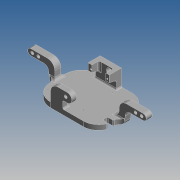
# Autodesk Inventor part: I006
Saved by Autodesk Inventor 2017 (Build 210142000, 142)
## iProperties
Created: 2018-10-19
Part Number: I006
Material: ABS
Document SubType Name: Modeling
Designer: Gilles Mottiez
Density: 1.06 g/cm^3
Appearance: Par défaut
Description: Plateforme mobile
Mass: 94.2161 g
Surface Area: 294.78 cm^2
Volume: 88.8831 cm^3
Author: Gilles Mottiez
Autodesk Inventor part; units mm, degrees
ref_plane "YZ Plane" through (0, 0, 0) normal (1, 0, 0) x (0, 1, 0)
ref_plane "XZ Plane" through (0, 0, 0) normal (0, 1, 0) x (-1, 0, 0)
ref_plane "XY Plane" through (0, 0, 0) normal (0, 0, 1) x (1, 0, 0)
sketch "Sketch1" plane through (0, 0, 0) normal (0, 0, 1) x (1, 0, 0)
  line L0 (0, 0) -> (106, 0)
  line L1 (106, 0) -> (106, -80)
  line L2 (106, -80) -> (0, -80)
  line L3 (0, -80) -> (0, 0)
  dimension "d0" = 106
  dimension "d1" = 80
  constraints: 8 end point, 2 parallel, 1 horizontal, 1 perpendicular
  measures "d0" distance of L0.start L0.end
  measures "d1" distance of L2.end L0.start
extrude "Extrusion1" add sketch "Sketch1" along normal blind 8
sketch "Esquisse2" plane through (0, 0, 8) normal (0, 0, 1) x (1, 0, 0)
  line L0 (106, 0) -> (0, 0) construction
  line L1 (0, 0) -> (0, -80) construction
  line L2 (0, -80) -> (106, -80) construction
  line L3 (106, -80) -> (106, 0) construction
  line L4 (8, -15.5) -> (66, -15.5) construction
  line L5 (66, -15.5) -> (66, -64.5) construction
  line L6 (66, -64.5) -> (8, -64.5) construction
  line L7 (8, -64.5) -> (8, -15.5) construction
  line L8 (0, -40) -> (106, -40) construction
  dimension "d4" = 58
  dimension "d5" = 49
  dimension "d6" = 8
  constraints: 10 end point, 4 coincident, 2 midpoint, 2 parallel, 1 horizontal, 1 perpendicular, 1 other
  measures "d4" distance of L4.start L4.end
  measures "d5" distance of L4.end L5.end
  measures "d6" distance between parallel lines of L1 L7
hole "Perçage1" at (8, -15.5, 8) at (8, -64.5, 8) at (66, -64.5, 8) at (66, -15.5, 8) direction (0, 0, -1) diameter 2 end through all
sketch "Esquisse3" plane through (106, -80, 0) normal (1, 0, 0) x (0, 0, -1)
  line L0 (0, 80) -> (0, 0) construction
  line L1 (0, 80) -> (-8, 80) construction
  line L2 (-8, 0) -> (-8, 80) construction
  line L3 (0, 0) -> (-8, 0) construction
  line L4 (-8, 40) -> (0, 40) construction
  line L5 (0, 45) -> (-33, 45)
  line L6 (-33, 45) -> (-33, 35)
  line L7 (-33, 35) -> (0, 35)
  line L8 (0, 35) -> (0, 45)
  dimension "d14" = 33
  dimension "d15" = 10
  constraints: 10 end point, 2 midpoint, 2 parallel, 1 horizontal, 1 perpendicular, 1 point on line, 1 other
  measures "d14" distance of L7.end L6.end
  measures "d15" distance of L5.end L6.end
extrude "Extrusion2" add sketch "Esquisse3" along normal blind 10
sketch "Esquisse4" plane through (0, -80, 0) normal (-1, 0, 0) x (0, 0, 1)
  line L0 (0, 0) -> (0, 80) construction
  line L1 (0, 0) -> (8, 0) construction
  line L2 (8, 80) -> (8, 0) construction
  line L3 (0, 80) -> (8, 80) construction
  line L4 (8, 40) -> (0, 40) construction
  line L5 (0, 45) -> (33, 45)
  line L6 (33, 45) -> (33, 35)
  line L7 (33, 35) -> (0, 35)
  line L8 (0, 35) -> (0, 45)
  dimension "d18" = 33
  dimension "d19" = 10
  constraints: 10 end point, 2 midpoint, 2 parallel, 1 horizontal, 1 perpendicular, 1 point on line, 1 other
  measures "d18" distance of L6.end L7.end
  measures "d19" distance of L5.end L6.end
extrude "Extrusion3" add sketch "Esquisse4" along normal blind 10
sketch "Esquisse5" plane through (-10, -80, 0) normal (-1, 0, 0) x (0, 0, 1)
  line L0 (33, 45) -> (0, 45) construction
  line L1 (0, 45) -> (0, 35) construction
  line L2 (0, 35) -> (33, 35) construction
  line L3 (33, 35) -> (33, 45) construction
  line L4 (33, 45) -> (23, 45)
  line L5 (23, 45) -> (23, 35)
  line L6 (23, 35) -> (33, 35)
  line L7 (33, 35) -> (33, 45)
  point P0 (0, 80)
  dimension "d22" = 10
  constraints: 8 end point, 2 parallel, 1 horizontal, 1 perpendicular, 1 point on line
  measures "d22" distance of L6.end L5.end
extrude "Extrusion4" add sketch "Esquisse5" along normal blind 34.5
sketch "Esquisse6" plane through (116, -80, 0) normal (1, 0, 0) x (0, 0, -1)
  line L0 (0, 45) -> (-33, 45) construction
  line L1 (-33, 45) -> (-33, 35) construction
  line L2 (-33, 35) -> (0, 35) construction
  line L3 (0, 35) -> (0, 45) construction
  line L4 (-33, 35) -> (-23, 35)
  line L5 (-23, 35) -> (-23, 45)
  line L6 (-23, 45) -> (-33, 45)
  line L7 (-33, 45) -> (-33, 35)
  point P0 (0, 80)
  dimension "d25" = 10
  constraints: 8 end point, 2 parallel, 1 horizontal, 1 perpendicular, 1 point on line
  measures "d25" distance of L6.end L5.end
extrude "Extrusion5" add sketch "Esquisse6" along normal blind 34.5
sketch "Esquisse7" plane through (0, -80, 0) normal (0, -1, 0) x (1, 0, 0)
  line L0 (106, 0) -> (0, 0) construction
  line L1 (106, 0) -> (106, 8) construction
  line L2 (0, 8) -> (106, 8) construction
  line L3 (0, 0) -> (0, 8) construction
  line L4 (53, 8) -> (53, 0) construction
  line L5 (28, 8) -> (63, 8) construction
  line L6 (63, 8) -> (63, 28) construction
  line L7 (63, 28) -> (28, 28) construction
  line L8 (28, 28) -> (28, 8) construction
  line L9 (28, 28) -> (28, 8)
  line L10 (63, 28) -> (63, 8)
  line L11 (28, 8) -> (63, 8)
  circle A0 centre (53, 28) radius 2.5
  line L12 (28, 28) -> (28, 35.5)
  line L13 (28, 35.5) -> (63, 35.5)
  line L14 (63, 35.5) -> (63, 28)
  line L15 (106, 0) -> (0, 0) construction
  point P0 (53, 0)
  point P1 (53, 0)
  dimension "d28" = 35
  dimension "d29" = 20
  dimension "d30" = 5
  dimension "d109" = 7.5
  dimension "d115" = 25
  constraints: 22 end point, 4 midpoint, 3 collinear, 3 perpendicular, 2 parallel, 2 point on line, 1 centre point, 1 horizontal, 1 vertical, 1 vertical alignment
  measures "d28" distance of L7.end L6.end
  measures "d29" distance of L6.end L5.end
  measures "d30" diameter of A0
  measures "d109" distance between parallel lines of L7 L13
  measures "d115" distance between parallel lines of L8 L4
extrude "Extrusion6" add sketch "Esquisse7" against normal blind 8
sketch "Esquisse8" plane through (0, 0, 0) normal (0, 1, 0) x (1, 0, 0)
  line L0 (0, 0) -> (106, 0) construction
  line L1 (0, 0) -> (0, -8) construction
  line L2 (106, -8) -> (0, -8) construction
  line L3 (106, 0) -> (106, -8) construction
  line L4 (53, -8) -> (53, 0) construction
  line L5 (64.8, -8) -> (29.8, -8) construction
  line L6 (29.8, -8) -> (29.8, -35) construction
  line L7 (29.8, -35) -> (64.8, -35) construction
  line L8 (64.8, -35) -> (64.8, -8) construction
  circle A0 centre (53, -28) radius 2.5 construction
  line L9 (28, -8) -> (28, -35.5) construction
  line L10 (63, -35.5) -> (63, -8) construction
  line L11 (28, -8) -> (63, -8) construction
  line L12 (58.8, -35) -> (35.8, -35) construction
  line L13 (35.8, -35) -> (35.8, -23) construction
  line L14 (35.8, -23) -> (58.8, -23) construction
  line L15 (58.8, -23) -> (58.8, -35) construction
  line L16 (47.3, -23) -> (47.3, -35) construction
  line L17 (64.8, -35) -> (29.8, -35)
  line L18 (29.8, -35) -> (29.8, -8)
  line L19 (29.8, -8) -> (64.8, -8)
  line L20 (64.8, -8) -> (64.8, -35)
  circle A1 centre (53, -28) radius 5
  line L21 (28, -35.5) -> (63, -35.5) construction
  dimension "d33" = 27
  dimension "d34" = 35
  dimension "d35" = 23
  dimension "d36" = 12
  dimension "d37" = 5.8
  dimension "d38" = 10
  constraints: 28 end point, 6 parallel, 4 midpoint, 3 horizontal, 3 perpendicular, 2 point on line, 1 centre point, 1 coincident, 1 other
  measures "d33" distance of L5.end L6.end
  measures "d34" distance of L6.end L7.end
  measures "d35" distance of L13.end L14.end
  measures "d36" distance of L12.end L13.end
  measures "d37" distance from line of A0.centre L15
  measures "d38" diameter of A1
extrude "Extrusion7" add sketch "Esquisse8" against normal blind 8
sketch "Esquisse9" plane through (0, -8, 0) normal (0, -1, 0) x (1, 0, 0)
  circle A0 centre (53, 28) radius 5 construction
  line L0 (0, 0) -> (106, 0) construction
  line L1 (0, 0) -> (0, 8) construction
  line L2 (29.8, 8) -> (0, 8) construction
  line L3 (29.8, 8) -> (29.8, 35) construction
  line L4 (29.8, 35) -> (64.8, 35) construction
  line L5 (64.8, 35) -> (64.8, 8) construction
  line L6 (106, 8) -> (64.8, 8) construction
  line L7 (106, 0) -> (106, 8) construction
  line L8 (53, 28) -> (29.8, 28) construction
  line L9 (36.2, 22) -> (29.8, 22) construction
  line L10 (29.8, 22) -> (29.8, 34) construction
  line L11 (29.8, 34) -> (36.2, 34) construction
  line L12 (36.2, 34) -> (36.2, 22) construction
  line L13 (64.8, 34) -> (59.2, 34) construction
  line L14 (59.2, 34) -> (59.2, 22) construction
  line L15 (59.2, 22) -> (64.8, 22) construction
  line L16 (64.8, 22) -> (64.8, 34) construction
  line L17 (29.8, 34) -> (36.2, 34) construction
  line L18 (36.2, 34) -> (36.2, 22) construction
  line L19 (36.2, 22) -> (29.8, 22) construction
  line L20 (29.8, 22) -> (29.8, 34) construction
  line L21 (59.2, 34) -> (64.8, 34) construction
  line L22 (64.8, 34) -> (64.8, 22) construction
  line L23 (64.8, 22) -> (59.2, 22) construction
  line L24 (59.2, 22) -> (59.2, 34) construction
  line L25 (29.8, 35) -> (36.2, 35)
  line L26 (36.2, 35) -> (36.2, 22)
  line L27 (36.2, 22) -> (29.8, 22)
  line L28 (29.8, 22) -> (29.8, 35)
  line L29 (64.8, 35) -> (59.2, 35)
  line L30 (59.2, 35) -> (59.2, 22)
  line L31 (59.2, 22) -> (64.8, 22)
  line L32 (64.8, 22) -> (64.8, 35)
  dimension "d41" = 12
  dimension "d42" = 23
  dimension "d43" = 6.2
  constraints: 50 end point, 12 parallel, 7 perpendicular, 6 horizontal, 3 point on line, 2 horizontal alignment, 1 other
  measures "d41" distance of L11.end L9.start
  measures "d42" distance between parallel lines of L12 L14
  measures "d43" distance from line of L8.start L14
extrude "Extrusion8" add sketch "Esquisse9" along normal blind 12
sketch "Esquisse10" plane through (106, -45, 8) normal (0, -1, 0) x (1, 0, 0)
  line L0 (0, 25) -> (0, 0) construction
  line L1 (0, -8) -> (0, 0) construction
  line L2 (0, -8) -> (10, -8) construction
  line L3 (10, 15) -> (10, -8) construction
  line L4 (10, 15) -> (44.5, 15) construction
  line L5 (44.5, 25) -> (44.5, 15) construction
  line L6 (0, 25) -> (44.5, 25) construction
  line L7 (44.5, 20) -> (0, 20) construction
  circle A0 centre (37, 20) radius 2.5
  circle A1 centre (27, 20) radius 2.5
  point P0 (-106, -8)
  dimension "d46" = 7.5
  dimension "d47" = 10
  dimension "d48" = 5
  dimension "d49" = 5
  constraints: 3 point on line, 2 centre point, 2 coincident, 2 end point, 1 midpoint, 1 parallel
  measures "d46" distance from line of L5 point (37, 20)
  measures "d47" distance of point (27, 20) point (37, 20)
  measures "d48" diameter of A0
  measures "d49" diameter of A1
extrude "Extrusion9" cut sketch "Esquisse10" against normal through all
sketch "Esquisse11" plane through (0, -45, 8) normal (0, -1, 0) x (1, 0, 0)
  line L0 (0, 25) -> (0, 0) construction
  line L1 (0, 25) -> (-44.5, 25) construction
  line L2 (-44.5, 15) -> (-44.5, 25) construction
  line L3 (-10, 15) -> (-44.5, 15) construction
  line L4 (-10, -8) -> (-10, 15) construction
  line L5 (0, -8) -> (-10, -8) construction
  line L6 (0, 0) -> (0, -8) construction
  line L7 (-44.5, 20) -> (0, 20) construction
  circle A0 centre (-37, 20) radius 2.5
  circle A1 centre (-27, 20) radius 2.5
  point P0 (0, -8)
  dimension "d52" = 5
  dimension "d53" = 5
  dimension "d54" = 7.5
  dimension "d55" = 10
  constraints: 3 point on line, 2 centre point, 2 end point, 1 midpoint, 1 perpendicular
  measures "d52" diameter of A0
  measures "d53" diameter of A1
  measures "d54" distance from line of L2 A0.centre
  measures "d55" distance of A1.centre A0.centre
extrude "Extrusion10" cut sketch "Esquisse11" against normal through all
fillet "Congé1" radius 5 4 edges at (150.5, -40, 33) (150.5, -40, 23) (-44.5, -40, 33) (-44.5, -40, 23)
sketch "Esquisse12" plane through (0, 0, 8) normal (0, 0, 1) x (1, 0, 0)
  line L0 (106, -80) -> (106, -45) construction
  line L1 (106, 0) -> (64.8, 0) construction
  line L2 (64.8, 0) -> (64.8, -8) construction
  line L3 (64.8, -8) -> (29.8, -8) construction
  line L4 (29.8, -8) -> (29.8, 0) construction
  line L5 (29.8, 0) -> (0, 0) construction
  line L6 (0, 0) -> (0, -35) construction
  line L7 (0, -80) -> (28, -80) construction
  line L8 (28, -80) -> (28, -72) construction
  line L9 (28, -72) -> (63, -72) construction
  line L10 (63, -72) -> (63, -80) construction
  line L11 (63, -80) -> (106, -80) construction
  circle A0 centre (66, -15.5) radius 1 construction
  circle A1 centre (8, -64.5) radius 1 construction
  circle A2 centre (8, -15.5) radius 1 construction
  circle A3 centre (66, -64.5) radius 1 construction
  line L12 (0, -35) -> (0, -45) construction
  line L13 (0, 0) -> (106, 0) construction
  line L14 (0, -35) -> (0, -45) projected
  line L15 (106, -45) -> (106, -35) projected
  line L16 (106, -35) -> (106, 0) projected
  line L17 (0, -45) -> (0, -80) projected
  point P0 (53, -40)
  point P1 (0, -40)
  point P2 (53, 0)
  constraints: 2 midpoint, 1 horizontal alignment, 1 vertical alignment
ref_plane "Plan de construction1" through (53, -40, 8) normal (0, 1, 0) x (1, 0, 0)
fillet "Congé11" radius 8 2 edges at (-10, -40, 23) (116, -40, 23)
fillet "Congé12" radius 3 2 edges at (33, -8, 22) (62, -8, 22)
fillet "Congé13" radius 3 2 edges at (36.2, -8, 20.5) (36.2, -8, 28.5)
fillet "Congé14" radius 1 2 edges at (59.2, -8, 28.5) (59.2, -8, 20.5)
fillet "Congé17" radius 12 2 edges at (0, -40, 33) (106, -40, 33)
chamfer "Chanfrein8" distance 2 distance2 9 1 edges at (33, -20, 22) measured on face at (33, -20, 22.5)
chamfer "Chanfrein9" distance 2 distance2 9 1 edges at (62, -20, 22) measured on face at (62, -20, 22.5)
chamfer "Chanfrein10" distance 15 distance2 2 1 edges at (-10, -40, 0) measured on face at (-10, -40, 0.5)
chamfer "Chanfrein11" distance 15 distance2 2 1 edges at (116, -40, 0) measured on face at (116, -40, 0.5)
fillet "Congé18" radius 7 2 edges at (-8.0001, -40, 0) (114.0001, -40, 0)
sketch "Esquisse13" plane through (28, -80, 35.5) normal (0, -1, 0) x (1, 0, 0)
  line L0 (-28, -27.5) -> (0, -27.5) construction
  line L1 (35, 0) -> (35, -27.5) construction
  line L2 (0, 0) -> (35, 0) construction
  line L3 (78, -35.5) -> (-28, -35.5) construction
  circle A0 centre (25, -7.5) radius 2.5 construction
  line L4 (30.425, -17.5) -> (23.175, -17.5) construction
  line L5 (23.175, -17.5) -> (23.175, -23.5) construction
  line L6 (23.175, -23.5) -> (30.425, -23.5) construction
  line L7 (30.425, -23.5) -> (30.425, -17.5) construction
  circle A1 centre (26.8, -20.5) radius 3 construction
  line L8 (35, -15) -> (20, -15)
  line L9 (20, -15) -> (20, -27.5)
  line L10 (20, -27.5) -> (35, -27.5)
  line L11 (35, -27.5) -> (35, -15)
  line L12 (0, -27.5) -> (0, 0) projected
  line L13 (78, -35.5) -> (78, -27.5) projected
  line L14 (35, -27.5) -> (78, -27.5) projected
  line L15 (-28, -35.5) -> (-28, -27.5) projected
  point P0 (-28, -35.5)
  point P1 (26.8, -17.5)
  point P2 (-14, -27.5)
  point P3 (30.425, -20.5)
  dimension "d110" = 7.25
  dimension "d111" = 6
  dimension "d113" = 1.8
  dimension "d114" = 6
  dimension "d118" = 4
  dimension "d119" = 15
  dimension "d120" = 12.5
  constraints: 16 end point, 4 parallel, 3 midpoint, 2 horizontal, 2 perpendicular, 1 centre point, 1 coincident, 1 horizontal alignment, 1 point on line, 1 vertical alignment
  measures "d110" distance of L6.end L5.end
  measures "d111" distance of L5.end L4.end
  measures "d113" horizontal distance of A0.centre A1.centre
  measures "d114" diameter of A1
  measures "d118" distance between parallel lines of L0 L6
  measures "d119" distance of L10.end L9.end
  measures "d120" distance of L9.end L8.end
extrude "Extrusion11" cut sketch "Esquisse13" against normal up to surface (8 mm away)
fillet "Congé19" radius 2 3 edges at (47.3, -8, 8) (64.8, -4, 8) (29.8, -4, 8)
fillet "Congé20" radius 2 3 edges at (28, -76, 8) (48, -76, 8) (38, -72, 8)
fillet "Congé21" radius 12 1 edges at (28, -76, 35.5)
fillet "Congé22" radius 7.5 2 edges at (63, -76, 35.5) (63, -76, 20.5)
fillet "Congé23" radius 2 1 edges at (48, -76, 20.5)
fillet "Congé24" radius 28 2 edges at (0, -80, 4) (0, 0, 4)
fillet "Congé25" radius 4 1 edges at (0, -40, 8)
sketch "Esquisse18" plane through (0, 0, 8) normal (0, 0, 1) x (1, 0, 0)
  line L0 (4, -45) -> (0, -45) construction
  line L1 (0, -45) -> (0, -52) construction
  arc A0 (0, -52) -> (26, -79.9285) centre (28, -52) ccw construction
  line L2 (26, -70) -> (26, -79.9285) construction
  line L3 (50, -70) -> (26, -70) construction
  line L4 (50, -80) -> (50, -70) construction
  line L5 (50, -80) -> (106, -80) construction
  line L6 (106, -80) -> (106, -45) construction
  line L7 (106, -45) -> (106, -35) construction
  line L8 (106, -35) -> (106, 0) construction
  line L9 (106, 0) -> (66.8, 0) construction
  line L10 (66.8, -10) -> (66.8, 0) construction
  line L11 (27.8, -10) -> (66.8, -10) construction
  line L12 (27.8, -0.0007) -> (27.8, -10) construction
  arc A1 (27.8, -0.0007) -> (0, -28) centre (28, -28) ccw construction
  line L13 (0, -28) -> (0, -35) construction
  line L14 (0, -35) -> (4, -35) construction
  line L15 (4, -45) -> (4, -35) construction
  circle A2 centre (66, -15.5) radius 1 construction
  circle A3 centre (8, -64.5) radius 1 construction
  circle A4 centre (8, -15.5) radius 1 construction
  circle A5 centre (66, -64.5) radius 1 construction
  line L16 (106, -16.5) -> (96, -16.5)
  line L17 (96, -16.5) -> (96, -24.5)
  line L18 (96, -24.5) -> (106, -24.5)
  line L19 (106, -24.5) -> (106, -16.5)
  line L20 (106, -62.5) -> (96, -62.5)
  line L21 (96, -62.5) -> (96, -54.5)
  line L22 (96, -54.5) -> (106, -54.5)
  line L23 (106, -54.5) -> (106, -62.5)
  line L24 (106, -40) -> (101, -40) construction
  point P0 (0, 0)
  dimension "d142" = 30
  dimension "d143" = 8
  dimension "d144" = 5
  dimension "d145" = 10
  constraints: 18 end point, 4 parallel, 3 horizontal, 2 midpoint, 2 perpendicular, 2 point on line, 1 collinear
  measures "d142" distance between parallel lines of L22 L18
  measures "d143" distance between parallel lines of L18 L16
  measures "d144" distance of L24.start L24.end
  measures "d145" distance of L16.start L16.end
extrude "Extrusion14" cut sketch "Esquisse18" against normal through all
fillet "Congé26" radius 25 2 edges at (106, -80, 4) (106, 0, 4)
fillet "Congé27" radius 2 8 edges at (106, -16.5, 4) (106, -62.5, 4) (96, -62.5, 4) (96, -54.5, 4) (106, -54.5, 4) (106, -24.5, 4) (96, -24.5, 4) (96, -16.5, 4)
fillet "Congé28" radius 9 4 edges at (106, -45, 4) (106, -35, 4) (0, -35, 4) (0, -45, 4)
fillet "Congé30" radius 4 2 edges at (-2.473, -45, 8) (-2.3998, -35, 8)
fillet "Congé31" radius 2 2 edges at (110.4486, -45, 8) (110.4943, -35, 8)
fillet "Congé32" radius 10 1 edges at (106, -40, 8)
sketch "Esquisse20" plane through (0, -20, 0) normal (0, -1, 0) x (1, 0, 0)
  circle A0 centre (53, 28) radius 5 construction
  line L0 (64.8, 10) -> (29.8, 10) construction
  line L1 (64.8, 10) -> (64.8, 19) construction
  line L2 (58.2, 19) -> (64.8, 19) construction
  line L3 (58.2, 35) -> (58.2, 19) construction
  line L4 (58.2, 35) -> (39.2, 35) construction
  line L5 (39.2, 19) -> (39.2, 35) construction
  line L6 (29.8, 19) -> (39.2, 19) construction
  line L7 (29.8, 19) -> (29.8, 10) construction
  line L8 (82.4894, 0) -> (82.4894, 8) construction
  line L9 (28, 0) -> (82.4894, 0) construction
  line L10 (28, 8.01) -> (28, 0) construction
  arc A1 (28, 8.01) -> (29.8, 10) centre (27.8, 10) ccw construction
  line L11 (29.8, 10) -> (29.8, 35) construction
  line L12 (29.8, 35) -> (64.8, 35) construction
  line L13 (64.8, 35) -> (64.8, 10) construction
  arc A2 (64.8, 10) -> (66.8, 8) centre (66.8, 10) ccw construction
  line L14 (82.4894, 8) -> (66.8, 8) construction
  circle A3 centre (53, 28) radius 5 construction
  line L15 (59.2, 21.2361) -> (59.2, 35) construction
  line L16 (36.2, 35) -> (36.2, 22) construction
  point P0 (0, 0)
  point P1 (61.5, 28)
  point P2 (34.5, 28)
  dimension "d155" = 8.5
  dimension "d156" = 27
  constraints: 2 horizontal alignment
  measures "d155" distance of point (61.5, 28) A0.centre
  measures "d156" distance of point (34.5, 28) point (61.5, 28)
hole "Perçage2" at (61.5, -20, 28) at (34.5, -20, 28) direction (0, 1, 0) diameter 2 end through all
